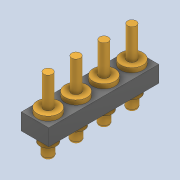
# Autodesk Inventor part: bat_conn_pin_
Saved by Autodesk Inventor 2020 (Build 240168000, 168)
## iProperties
Created: 2021-08-25
Part Number: bat_conn_pin_
Material: Generic
Document SubType Name: Modeling
Designer: Shuang Peng
Density: 1 g/cm^3
Appearance: Default
Author: Shuang Peng
Autodesk Inventor part; units mm, degrees
ref_plane "YZ Plane" through (0, 0, 0) normal (1, 0, 0) x (0, 1, 0)
ref_plane "XZ Plane" through (0, 0, 0) normal (0, 1, 0) x (-1, 0, 0)
ref_plane "XY Plane" through (0, 0, 0) normal (0, 0, 1) x (1, 0, 0)
sketch "Sketch1" plane through (0, 0, 0) normal (0, 1, 0) x (-1, 0, 0)
  line L0 (1.25, 5) -> (-1.25, 5)
  line L1 (-1.25, 5) -> (-1.25, -5)
  line L2 (-1.25, -5) -> (1.25, -5)
  line L3 (1.25, -5) -> (1.25, 5)
  line L4 (1.25, 5) -> (-1.25, -5) construction
  line L5 (-1.25, 5) -> (1.25, -5) construction
  point P0 (0, 0)
  dimension "d0" = 2.5
  dimension "d1" = 10
  constraints: 12 end point, 2 midpoint, 2 parallel, 1 horizontal, 1 perpendicular
  measures "d0" distance of L0.start L0.end
  measures "d1" distance of L1.end L0.end
extrude "Extrusion1" add sketch "Sketch1" along normal blind 1.5
sketch "Sketch2" plane through (0, 1.5, 0) normal (0, 1, 0) x (1, 0, 0)
  line L0 (0, 0) -> (0, 3.81)
  circle A0 centre (0, 3.81) radius 1
  dimension "d4" = 3.81
  dimension "d5" = 2
  constraints: 2 end point, 1 centre point, 1 coincident, 1 vertical
  measures "d4" distance of L0.start L0.end
  measures "d5" diameter of A0
extrude "Extrusion2" add sketch "Sketch2" along normal blind 0.4
sketch "Sketch3" plane through (0, 1.5, 0) normal (0, 1, 0) x (1, 0, 0)
  circle A0 centre (0, 3.81) radius 1 projected
  circle A1 centre (0, 3.81) radius 0.4
  point P0 (0, 0)
  dimension "d8" = 0.8
  constraints: 1 centre point, 1 coincident
  measures "d8" diameter of A1
extrude "Extrusion3" add sketch "Sketch3" along normal blind 3.2 contours A1
sketch "Sketch4" plane through (0, 0, 0) normal (0, -1, 0) x (1, 0, 0)
  circle A0 centre (0, -3.81) radius 1 projected
  circle A1 centre (0, -3.81) radius 0.75
  point P0 (0, 0)
  dimension "d11" = 1.5
  constraints: 1 centre point, 1 coincident
  measures "d11" diameter of A1
extrude "Extrusion4" add sketch "Sketch4" along normal blind 0.8 contours A1
sketch "Sketch5" plane through (0, 0, 0) normal (0, -1, 0) x (1, 0, 0)
  circle A0 centre (0, -3.81) radius 0.75 projected
  circle A1 centre (0, -3.81) radius 0.475
  point P0 (0, 0)
  dimension "d14" = 0.95
  constraints: 1 centre point, 1 coincident
  measures "d14" diameter of A1
extrude "Extrusion5" add sketch "Sketch5" along normal blind 2 contours A1
fillet "Fillet1" radius 0.25 1 edges at (-0.475, -2, -3.81)
pattern_linear "Rectangular Pattern1" count 4 spacing 2.54 along (0, 0, 1) of "Extrusion2", "Extrusion3", "Extrusion4", "Extrusion5", "Fillet1"
body "Solid1"
